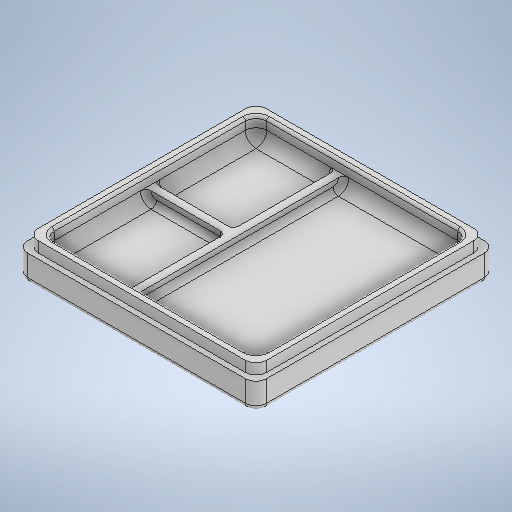
# Autodesk Inventor part: box-1
Saved by Autodesk Inventor 2025 (Build 290162000, 162)
## iProperties
Created: 2026-01-27
Part Number: box-1
Material: 一般
Document SubType Name: Modeling
Designer: mahhy
Density: 1 g/cm^3
Appearance: 既定
Author: mahhy
## iProperties of the stored document box-1_3D プリント.ipt
Created: 2026-01-27
Part Number: box-1_3D プリント
Material: 一般
Document SubType Name: Modeling
Designer: mahhy
Density: 1 g/cm^3
Appearance: 既定
Author: mahhy
Autodesk Inventor part; units mm, degrees
ref_plane "YZ Plane" through (0, 0, 0) normal (1, 0, 0) x (0, 1, 0)
ref_plane "XZ Plane" through (0, 0, 0) normal (0, 1, 0) x (-1, 0, 0)
ref_plane "XY Plane" through (0, 0, 0) normal (0, 0, 1) x (1, 0, 0)
sketch "底面スケッチ" plane through (0, 0, 0) normal (0, 1, 0) x (-1, 0, 0)
  line L0 (-2, 0) -> (-43, 0)
  line L1 (-45, -2) -> (-45, -43)
  line L2 (-43, -45) -> (-2, -45)
  line L3 (0, -43) -> (0, -2)
  arc A0 (-2, -45) -> (0, -43) centre (-2, -43) ccw
  arc A1 (-45, -43) -> (-43, -45) centre (-43, -43) ccw
  arc A2 (0, -2) -> (-2, 0) centre (-2, -2) ccw
  arc A3 (-43, 0) -> (-45, -2) centre (-43, -2) ccw
  point P0 (0, 0)
  point P1 (-45, -45)
  point P2 (-45, 0)
  point P3 (0, -45)
  dimension "d2" = 45
  dimension "d3" = 45
  dimension "d18" = 2
  constraints: 8 end point, 8 point on circle, 8 point on line, 8 tangent, 4 centre point, 3 equal radius, 2 parallel, 1 horizontal, 1 perpendicular
  measures "d2" distance of point (0, -45) point (-45, -45)
  measures "d3" distance of point (-45, -45) point (-45, 0)
  measures "d18" radius of A0
extrude "押し出し1" add sketch "底面スケッチ" along normal blind 3
sketch "スケッチ3" plane through (0, 3, 0) normal (0, 1, 0) x (1, 0, 0)
  line L0 (4.5, 42.5) -> (40.5, 42.5)
  line L1 (42.5, 40.5) -> (42.5, 4.5)
  line L2 (40.5, 2.5) -> (4.5, 2.5)
  line L3 (2.5, 4.5) -> (2.5, 40.5)
  line L4 (43, 45) -> (2, 45) projected
  line L5 (0, 0) -> (43, 0) projected
  line L6 (0, 43) -> (0, 0) projected
  line L7 (45, 2) -> (45, 43) projected
  arc A0 (0, 2) -> (2, 0) centre (2, 2) ccw projected
  arc A1 (43, 0) -> (45, 2) centre (43, 2) ccw projected
  arc A2 (45, 43) -> (43, 45) centre (43, 43) ccw projected
  arc A3 (2, 45) -> (0, 43) centre (2, 43) ccw projected
  arc A4 (4.5, 42.5) -> (2.5, 40.5) centre (4.5, 40.5) ccw
  arc A5 (2.5, 4.5) -> (4.5, 2.5) centre (4.5, 4.5) ccw
  arc A6 (40.5, 2.5) -> (42.5, 4.5) centre (40.5, 4.5) ccw
  arc A7 (42.5, 40.5) -> (40.5, 42.5) centre (40.5, 40.5) ccw
  point P0 (2.5, 42.5)
  point P1 (42.5, 2.5)
  point P2 (42.5, 42.5)
  point P3 (2.5, 2.5)
  point P4 (40, 40)
  point P5 (40, 0)
  dimension "d12" = 2.5
  dimension "d13" = 2.5
  dimension "d14" = 2.5
  dimension "d15" = 2.5
  dimension "d19" = 2
  constraints: 8 end point, 8 point on circle, 8 point on line, 8 tangent, 4 centre point, 3 equal radius, 2 parallel, 1 horizontal, 1 perpendicular, 2 other
  measures "d13" distance between parallel lines of L5 L2
  measures "d14" distance between parallel lines of L6 L3
  measures "d19" radius of A4
extrude "押し出し3" add sketch "スケッチ3" along normal blind 4 contours A2 L7 A1 L5 A0 L6 A3 L4
sketch "スケッチ4" plane through (0, 3, 0) normal (0, 1, 0) x (1, 0, 0)
  line L0 (4.5, 42.5) -> (40.5, 42.5) projected
  line L1 (4.5, 2.5) -> (40.5, 2.5) projected
  line L2 (17.5, 42.5) -> (19, 42.5)
  line L3 (19, 42.5) -> (19, 2.5)
  line L4 (19, 2.5) -> (17.5, 2.5)
  line L5 (17.5, 2.5) -> (17.5, 42.5)
  line L6 (2.5, 4.5) -> (2.5, 40.5) projected
  line L7 (2.5, 23.25) -> (17.5, 23.25)
  line L8 (17.5, 23.25) -> (17.5, 21.75)
  line L9 (17.5, 21.75) -> (2.5, 21.75)
  line L10 (2.5, 21.75) -> (2.5, 23.25)
  line L11 (0, 43) -> (0, 2) projected
  point P0 (0, 0)
  point P1 (2.5, 22.5)
  point P2 (0, 22.5)
  point P3 (17.5, 21.75)
  point P4 (2.5, 21.75)
  dimension "d20" = 1.5
  dimension "d21" = 15
  dimension "d22" = 1.5
  constraints: 16 end point, 4 parallel, 4 point on line, 2 horizontal, 2 midpoint, 2 perpendicular, 1 horizontal alignment
  measures "d20" distance of L3.end L4.end
  measures "d21" distance between parallel lines of L6 L5
  measures "d22" distance of L7.end L8.end
extrude "押し出し4" add sketch "スケッチ4" along normal blind 2
fillet "フィレット1" radius 2 11 edges at (41.9142, 3, -3.0858) (42.5, 3, -22.5) (41.9142, 3, -41.9142) (29.75, 3, -42.5) (29.75, 3, -2.5) (3.0858, 3, -3.0858) (2.5, 3, -13.125) (11, 3, -2.5) (3.0858, 3, -41.9142) (11, 3, -42.5) (2.5, 3, -31.875)
fillet "フィレット2" radius 1 11 edges at (19, 3.5858, -3.0858) (19, 3.5858, -41.9142) (19, 3, -22.5) (3.0858, 3.5858, -21.75) (11, 3, -21.75) (3.0858, 3.5858, -23.25) (11, 3, -23.25) (17.5, 3.5858, -41.9142) (17.5, 3, -31.875) (17.5, 3.5858, -3.0858) (17.5, 3, -13.125)
sketch "スケッチ5" plane through (0, 7, 0) normal (0, 1, 0) x (1, 0, 0)
  line L0 (3, 1) -> (42, 1)
  line L1 (44, 3) -> (44, 42)
  line L2 (42, 44) -> (3, 44)
  line L3 (1, 42) -> (1, 3)
  line L4 (0, 43) -> (0, 2) projected
  line L5 (45, 2) -> (45, 43) projected
  line L6 (2, 0) -> (43, 0) projected
  line L7 (43, 45) -> (2, 45) projected
  arc A0 (1, 3) -> (3, 1) centre (3, 3) ccw
  arc A1 (42, 1) -> (44, 3) centre (42, 3) ccw
  arc A2 (44, 42) -> (42, 44) centre (42, 42) ccw
  arc A3 (3, 44) -> (1, 42) centre (3, 42) ccw
  arc A4 (43, 0) -> (45, 2) centre (43, 2) ccw projected
  arc A5 (45, 43) -> (43, 45) centre (43, 43) ccw projected
  arc A6 (2, 45) -> (0, 43) centre (2, 43) ccw projected
  arc A7 (0, 2) -> (2, 0) centre (2, 2) ccw projected
  point P0 (0, 0)
  dimension "d27" = 1
  dimension "d28" = 1
  dimension "d29" = 1
  dimension "d30" = 1
  dimension "d31" = 2
  dimension "d32" = 2
  dimension "d33" = 2
  dimension "d34" = 2
  constraints: 8 end point, 8 point on circle, 8 tangent, 4 centre point, 2 parallel, 1 horizontal, 1 perpendicular
  measures "d27" distance between parallel lines of L4 L3
  measures "d28" distance between parallel lines of L5 L1
  measures "d29" distance between parallel lines of L0 L6
  measures "d30" distance between parallel lines of L7 L2
  measures "d31" radius of A0
  measures "d32" radius of A1
  measures "d33" radius of A2
  measures "d34" radius of A3
extrude "押し出し5" cut sketch "スケッチ5" against normal blind 2
fillet "フィレット3" radius 1 4 edges at (17.2071, 3.2929, -23.5429) (17.5, 4.5, -23.25) (17.2071, 3.2929, -21.4571) (17.5, 4.5, -21.75)
fillet "フィレット4" radius 1 8 edges at (44.4142, 0, -44.4142) (22.5, 0, -45) (0.5858, 0, -44.4142) (0, 0, -22.5) (0.5858, 0, -0.5858) (22.5, 0, 0) (44.4142, 0, -0.5858) (45, 0, -22.5)
fillet "フィレット5" radius 0.5 8 edges at (41.9142, 7, -41.9142) (42.5, 7, -22.5) (41.9142, 7, -3.0858) (22.5, 7, -2.5) (3.0858, 7, -3.0858) (2.5, 7, -22.5) (3.0858, 7, -41.9142) (22.5, 7, -42.5)
sketch "スケッチ6" plane through (0, 0, 0) normal (0, -1, 0) x (1, 0, 0)
  line L0 (2, -1) -> (43, -1) projected
  line L1 (44, -2) -> (44, -43) projected
  circle A0 centre (22.5, -22.5) radius 12.5
  point P0 (0, 0)
  point P1 (22.5, -1)
  point P2 (44, -22.5)
  point P3 (22.5, -1)
  point P4 (44, -22.5)
  dimension "d41" = 25
  constraints: 4 midpoint, 1 centre point, 1 horizontal alignment, 1 vertical alignment
  measures "d41" diameter of A0
extrude "押し出し6" cut sketch "スケッチ6" against normal blind 2.5
equation "\"d3\" = d2"
equation "\"d22\" = d20"
equation "\"d28\" = d27"
equation "\"d29\" = d27"
equation "\"d30\" = d27"
